screw_wheel_27_m4 (Autodesk Fusion 360 design; units mm, degrees)
Autodesk Fusion 360 part; units mm, degrees
note: some values were not read from the file. Set by a fixed rule: which sketch regions a step uses.
sketch "Sketch1" plane through (0, 0, 0) normal (0, 1, 0) x (1, 0, 0)
  circle A0 centre (0, 0) radius 13.5
  circle A1 centre (0, 0) radius 2.1
  dimension "d1" = 27
  dimension "d2" = 4.2
  constraint coincident A0.centre A1.centre
  constraint concentric A0 A1
  measures "d1" diameter of A0
  measures "d2" diameter of A1
extrude "Extrude1" add sketch "Sketch1" along normal blind 4
fillet "Fillet1" radius 1 2 edges at (-12.586419, 0, 4.881808) (-12.586419, 4, 4.881808)
sketch "Sketch2" plane through (0, 0, 0) normal (0, -1, 0) x (1, 0, 0)
  circle A0 centre (0, 0) radius 2.1
  circle A1 centre (0, 0) radius 12.5
  circle A2 centre (0, 0) radius 13.5
  circle A3 centre (0, 13.5) radius 0.75
  circle A4 centre (-1.180917, 12.845833) radius 0.6
  circle A5 centre (1.180917, 12.845833) radius 0.6
  dimension "d7" = 1.5
  dimension "d8" = 1.2
  constraint coincident A2 A3.centre
  constraint vertical A0.centre A3.centre
  constraint tangent A2 A4
  constraint tangent A3 A4
  constraint tangent A3 A5
  constraint tangent A2 A5
  constraint equal A4 A5
  measures "d7" diameter of A3
  measures "d8" diameter of A4
extrude "Extrude2" cut sketch "Sketch2" against normal through all contours A2 A3 A4 | A2 A3 | A2 A3 A5 picked at (-0.853978, 13.441505) picked at (-0.017734, 13.249086) picked at (0.853978, 13.441505)
pattern_circular "C-Pattern1" count 30 over 360 about axis through (0, 1.75, 0) along (0, 1, 0) of "Extrude2"
sketch "Sketch3" plane through (0, 0, 0) normal (0, -1, 0) x (1, 0, 0)
  circle A0 centre (0, 0) radius 2.1
  circle A1 centre (0, 0) radius 12.5
  line L0 (-2.078461, 3.6) -> (-4.156922, 0)
  line L1 (-4.156922, 0) -> (-2.078461, -3.6)
  line L2 (-2.078461, -3.6) -> (2.078461, -3.6)
  line L3 (2.078461, -3.6) -> (4.156922, 0)
  line L4 (4.156922, 0) -> (2.078461, 3.6)
  line L5 (2.078461, 3.6) -> (-2.078461, 3.6)
  dimension "d12" = 7.2
  constraint coincident A0.centre A1.centre
  measures "d12" distance of L2 L5
extrude "Extrude3" cut sketch "Sketch3" against normal blind 3.5 contours L0 L1 L2 L3 L4 L5 picked at (0.052311, -3.098043)
